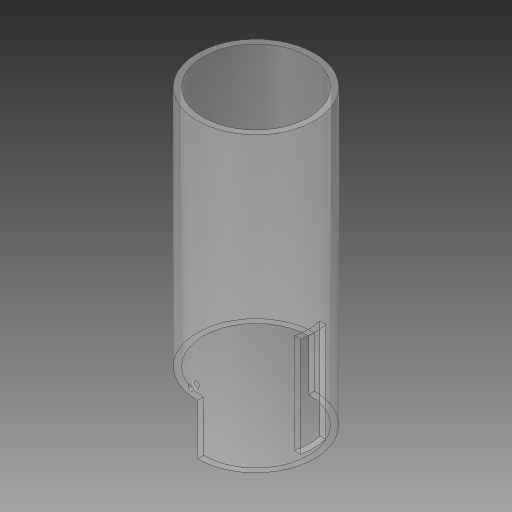
# Autodesk Inventor part: cylindre-lanceur
Saved by Autodesk Inventor 2019 (Build 230136000, 136)
## iProperties
Created: 2018-01-27
Part Number: cylindre-lanceur
Material: Générique
Document SubType Name: Modeling
Designer: franc
Density: 1 g/cm^3
Appearance: Polycarbonate - Transparent
Author: franc
Autodesk Inventor part; units mm, degrees
ref_plane "XZ Plane" through (0, 0, 0) normal (0, 1, 0) x (-1, 0, 0)
sketch "Esquisse1" plane through (0, 0, 0) normal (0, 1, 0) x (-1, 0, 0)
  circle A0 centre (0, 0) radius 27
  circle A1 centre (0, 0) radius 30
  dimension "d0" = 60
  dimension "d1" = 54
  constraints: 2 centre point, 2 coincident
  measures "d0" diameter of A1
  measures "d1" diameter of A0
extrude "Extrusion1" add sketch "Esquisse1" along normal blind 150
ref_plane "Plan de construction1" through (30, 0, 0) normal (1, 0, 0) x (0, 1, 0)
sketch "Esquisse2" plane through (30, 0, 0) normal (1, 0, 0) x (0, 1, 0)
  line L0 (56, 6.5) -> (5, 6.5)
  line L1 (5, 6.5) -> (5, -6.5)
  line L2 (5, -6.5) -> (56, -6.5)
  line L3 (56, -6.5) -> (56, 6.5)
  line L4 (0, -27) -> (0, 27) projected
  line L5 (-11.2, 0) -> (67.2, 0) projected
  point P0 (0, 0)
  dimension "d5" = 5
  dimension "d6" = 51
  dimension "d7" = 13
  dimension "d8" = 6.5
  constraints: 8 end point, 2 parallel, 1 horizontal, 1 perpendicular
  measures "d5" distance between parallel lines of L4 L1
  measures "d6" distance of L0.start L0.end
  measures "d7" distance of L2.end L0.start
  measures "d8" distance between parallel lines of L5 L0
extrude "Extrusion2" cut sketch "Esquisse2" against normal blind 10
sketch "Esquisse3" plane through (0, 0, 0) normal (0, -1, 0) x (1, 0, 0)
  circle A0 centre (0, 0) radius 27 projected
  arc A1 (0, 27) -> (0, -27) centre (0, 0) ccw
  circle A2 centre (0, 0) radius 30 projected
  arc A3 (0, 30) -> (0, -30) centre (0, 0) ccw
  line L0 (0, 30) -> (0, 27)
  line L1 (0, -30) -> (0, -27)
  constraints: 4 end point, 4 point on circle, 2 centre point, 2 vertical alignment, 1 coincident, 1 collinear, 1 vertical, 2 other
extrude "Extrusion3" cut sketch "Esquisse3" against normal blind 26 contours A0 L1 A2 L0 picked at (-4.547, -28.4479)
ref_plane "Work Plane2" through (0, 0, 30) normal (0, 0, 1) x (1, 0, 0)
sketch "Sketch4" plane through (0, 0, 30) normal (0, 0, 1) x (1, 0, 0)
  circle A0 centre (-3.6258, 29.618) radius 1.5 projected
  point P0 (0, 0)
extrude "Extrusion4" cut sketch "Sketch4" against normal up to next
